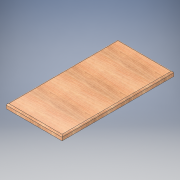
# Autodesk Inventor part: Part1
Saved by Autodesk Inventor 2017 (Build 210142000, 142)
## iProperties
Created: 2019-01-25
Part Number: Part1
Material: Generic
Document SubType Name: Modeling
Designer: Cj Lohnes
Density: 1 g/cm^3
Appearance: Default
Author: Cj Lohnes
Autodesk Inventor part; units mm, degrees
ref_plane "YZ Plane" through (0, 0, 0) normal (1, 0, 0) x (0, 1, 0)
ref_plane "XZ Plane" through (0, 0, 0) normal (0, 1, 0) x (-1, 0, 0)
ref_plane "XY Plane" through (0, 0, 0) normal (0, 0, 1) x (1, 0, 0)
sketch "Sketch1" plane through (0, 0, 0) normal (0, 1, 0) x (-1, 0, 0)
  line L0 (3544.3132, 6836.0134) -> (369.3132, 6836.0134)
  line L1 (369.3132, 6836.0134) -> (369.3132, 486.0134)
  line L2 (369.3132, 486.0134) -> (3544.3132, 486.0134)
  line L3 (3544.3132, 486.0134) -> (3544.3132, 6836.0134)
  point P0 (0, 0)
  dimension "d0" = 6350
  dimension "d1" = 3175
  constraints: 8 end point, 2 parallel, 1 horizontal, 1 perpendicular
  measures "d0" distance of L2.end L0.start
  measures "d1" distance of L1.end L2.end
extrude "Extrusion1" add sketch "Sketch1" along normal blind 254
fillet "Fillet1" radius 76.2 4 edges at (-3544.3132, 254, 3661.0134) (-1956.8132, 254, 486.0134) (-369.3132, 254, 3661.0134) (-1956.8132, 254, 6836.0134)
sketch "Sketch2" plane through (0, 0, 0) normal (0, -1, 0) x (1, 0, 0)
  circle A0 centre (-623.3132, 6582.0134) radius 190.5
  line L0 (-3544.3132, 6836.0134) -> (-369.3132, 6836.0134) projected
  line L1 (-369.3132, 6836.0134) -> (-369.3132, 486.0134) projected
  line L2 (-369.3132, 6836.0134) -> (-369.3132, 486.0134) projected
  line L3 (-369.3132, 3661.0134) -> (-3544.3132, 3661.0134)
  line L4 (-3544.3132, 486.0134) -> (-3544.3132, 6836.0134) projected
  line L5 (-369.3132, 486.0134) -> (-3544.3132, 486.0134) projected
  line L6 (-1956.8132, 486.0134) -> (-1956.8132, 6836.0134)
  circle A1 centre (-623.3132, 740.0134) radius 190.5
  circle A2 centre (-3290.3132, 6582.0134) radius 190.5
  line L7 (-3544.3132, 6836.0134) -> (-3544.3132, 486.0134)
  circle A3 centre (-3290.3132, 740.0134) radius 190.5
  point P0 (0, 0)
  dimension "d4" = 381
  dimension "d5" = 254
  dimension "d6" = 254
  constraints: 6 end point, 4 centre point, 4 midpoint, 3 symmetric about line, 3 other
  measures "d4" diameter of A0
  measures "d5" distance from line of L0 A0.centre
  measures "d6" distance from line of L1 A0.centre
extrude "Extrusion2" cut sketch "Sketch2" against normal blind 88.9 contours A0
equation "\"d1\" = 0.5 * d0"
equation "\"d6\" = d5"
body "Solid1"
